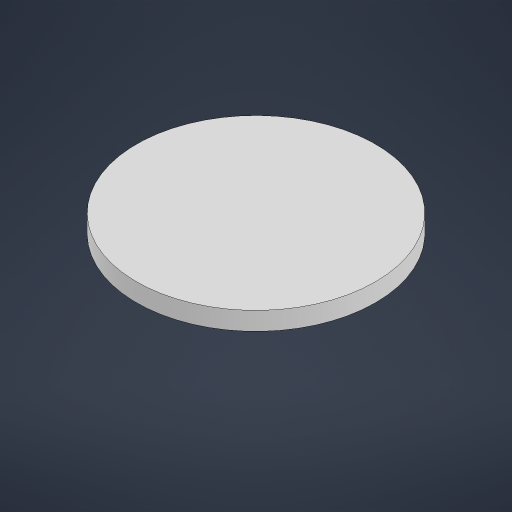
# Autodesk Inventor part: COne_mirror
Saved by Autodesk Inventor 2024.2 (Build 282272000, 272)
## iProperties
Created: 2024-02-16
Part Number: COne_mirror
Material: 一般
Document SubType Name: Modeling
Designer: Hanaoka
Density: 1 g/cm^3
Appearance: 既定
Author: Hanaoka
Autodesk Inventor part; units mm, degrees
ref_plane "YZ Plane" through (0, 0, 0) normal (1, 0, 0) x (0, 1, 0)
ref_plane "XZ Plane" through (0, 0, 0) normal (0, 1, 0) x (-1, 0, 0)
ref_plane "XY Plane" through (0, 0, 0) normal (0, 0, 1) x (1, 0, 0)
sketch "スケッチ1" plane through (0, 0, 0) normal (0, 0, 1) x (1, 0, 0)
  line L0 (2, 1.1547) -> (22.6, 13.0481)
  line L1 (22.6, 13.0481) -> (-22.6, 13.0481)
  line L2 (-22.6, 13.0481) -> (-2, 1.1547)
  line L3 (-22.6, 13.0481) -> (-22.6, 15.0481)
  line L4 (-22.6, 15.0481) -> (-24.8, 15.0481)
  line L5 (-24.8, 15.0481) -> (-24.8, 13.0481)
  line L6 (-24.8, 13.0481) -> (-26.3, 13.0481)
  line L7 (-26.3, 13.0481) -> (-26.3, 17.0481)
  line L8 (-26.3, 17.0481) -> (26.3, 17.0481)
  line L9 (26.3, 17.0481) -> (26.3, 13.0481)
  line L10 (26.3, 13.0481) -> (24.8, 13.0481)
  line L11 (24.8, 13.0481) -> (24.8, 15.0481)
  line L12 (24.8, 15.0481) -> (22.6, 15.0481)
  line L13 (22.6, 15.0481) -> (22.6, 13.0481)
  line L14 (-22.6, 15.0481) -> (-22.6, 55.0481)
  line L15 (-22.6, 55.0481) -> (22.6, 55.0481)
  line L16 (22.6, 55.0481) -> (22.6, 15.0481)
  arc A0 (-2, 1.1547) -> (2, 1.1547) centre (0, 4.6188) ccw
  line L17 (0, 0) -> (0, 55.0481)
  point P0 (0, 0.6188)
  point P1 (0, 17.0481)
  dimension "d0" = 45.2
  dimension "d1" = 30
  dimension "d2" = 2.2
  dimension "d3" = 1.5
  dimension "d4" = 2
  dimension "d5" = 4
  dimension "d6" = 40
  dimension "d7" = 4
  constraints: 36 end point, 11 perpendicular, 4 equal length, 4 point on line, 2 point on circle, 2 tangent, 2 vertical, 1 centre point, 1 collinear, 1 horizontal, 1 midpoint
  measures "d0" distance of L0.end L1.end
  measures "d1" angle of L0 L1
  measures "d2" distance of L3.end L4.end
  measures "d3" distance of L5.end L6.end
  measures "d4" distance of L1.end L3.end
  measures "d5" distance of L6.end L7.end
  measures "d6" distance of L15.end L12.end
  measures "d7" radius of A0
revolve "回転1" add sketch "スケッチ1" angle 360 about axis through (0, 0, 0) along (0, 1, 0) contours A0 L17 L1 L0 | L1 L17 L8 L16 L13 | L16 L8 L9 L10 L11 L12
